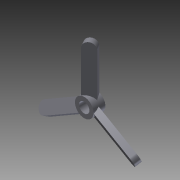
# Autodesk Inventor part: LEGO Brick 2421
Saved by Autodesk Inventor 2011 SP1 (Build 150282100, 282)
## iProperties
Company: Allseas Engineering BV
Created: 2011-09-28
Part Number: LEGO Brick 2421
Cost Center: 0 kg
Material: Steel
Document SubType Name: Modeling
Designer: BvH
Authority: 0 mm^3
Stock Number: =<Filenr>_<Document number>
Density: 7.85 g/cm^3
Act. Code: DW000
SaveDate: 2011-07-28
SaveTime: 18:32
FileName: Standard
TotalMass: 0 kg
TotalVolume: 0 mm^3
Subject: =<Title><TITLE 1_2> <TITLE 2_2>
Author: BvH
Autodesk Inventor part; units mm, degrees
ref_plane "YZ Plane" through (0, 0, 0) normal (1, 0, 0) x (0, 1, 0)
ref_plane "XZ Plane" through (0, 0, 0) normal (0, 1, 0) x (-1, 0, 0)
ref_plane "XY Plane" through (0, 0, 0) normal (0, 0, 1) x (1, 0, 0)
sketch "Sketch2" plane through (0, 0, 0) normal (0, 1, 0) x (-1, 0, 0)
  circle A0 centre (0, 0) radius 2.5
  circle A1 centre (0, 0) radius 1.4
  dimension "d9" = 5
  dimension "d10" = 2.8
  constraints: 2 centre point, 2 coincident
  measures "d9" diameter of A0
  measures "d10" diameter of A1
sketch "Sketch1" plane through (0, 0, 0) normal (0, 0, 1) x (1, 0, 0)
  line L0 (-1.7856, -0.1072) -> (0.9856, 1.4928)
  line L1 (0.9856, 1.4928) -> (1.7856, 0.1072)
  line L2 (1.7856, 0.1072) -> (-0.9856, -1.4928)
  line L3 (-0.9856, -1.4928) -> (-1.7856, -0.1072)
  line L4 (0.9856, 1.4928) -> (-0.9856, -1.4928) construction
  line L5 (0, -2.0899) -> (0, 2.0899) construction
  line L6 (-2.4999, 0) -> (2.4999, 0) construction
  point P0 (0, 0)
  dimension "d0" = 1.6
  dimension "d1" = 3.2
  dimension "d2" = 30
  constraints: 10 end point, 3 midpoint, 2 parallel, 1 perpendicular
  measures "d0" distance between parallel lines of L2 L0
  measures "d1" distance between parallel lines of L3 L1
  measures "d2" angle of L2 L6
extrude "Extrusion1" add sketch "Sketch1" along normal blind 15
fillet "Fillet1" radius 1.6 2 edges at (1.3856, 0.8, 15) (-1.3856, -0.8, 15)
pattern_circular "Circular Pattern1" count 3 over 360 about axis through (0, -10, 0) along (0, 1, 0) of "Extrusion1", "Fillet1"
extrude "Extrusion2" add sketch "Sketch2" along normal mid plane 3.2 contours A0 | A1
extrude "Extrusion3" cut sketch "Sketch2" along normal through all both and the other way through all contours A1
equation "\"d5\" = 0.5 * d1"
body "Solid1"
